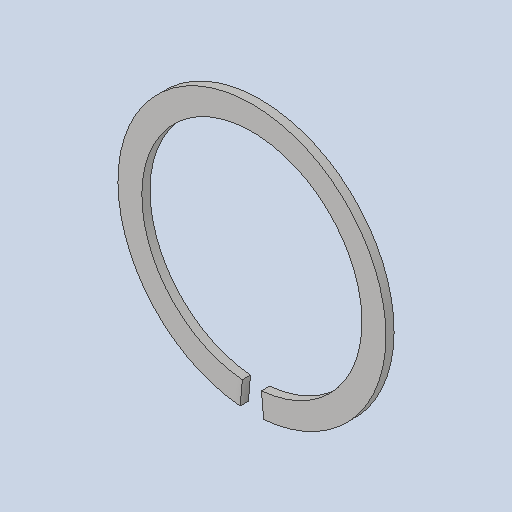
# Autodesk Inventor part: RING-6201ZZ
Saved by Autodesk Inventor 2025.1 (Build 291241000, 241)
## iProperties
Created: 2023-12-27
Part Number: RING-6201ZZ
Material: Generic
Catalog Web Link: www.cadenas.de
Description: RING-External Retaining Ring
Vendor: MISUMI
Document SubType Name: Modeling
Designer: psAdmin
Manufacturer: MISUMI
Mass: 0.374469 g
Surface Area: 9.04715 cm^2
Volume: 0.374469 cm^3
Density: 1 g/cm^3
Appearance: PSOLRGB-175-175-175
Category: PARTsolutions
Company: MISUMI
PSOL_IDENT_0: {$CADENAS_DATA/23d-libs/misumi/metric/12_bearing_holders/sb6905zznr_ring.prj},160 {VTYP=3D},{NB=RING
PSOL_IDENT_1: -6201ZZ},{LINA=RING-6201ZZ},{NN=RING},{DATE=25.04.2017 02:57:49},{GEOMDATE=03.07.2009 00:00:00},{VER
PSOL_IDENT_2: SION=},{LINEID=90},{WBVAR=},{WBNUMERIC=}  {NB=RING-6201ZZ},{LINA=RING-6201ZZ},{KT=DUMMY},{PN=RING-62
PSOL_IDENT_3: 01ZZ},{BN=6201ZZ},{D1=36.7},{FF=1.120},{D=30.150}
NB: RING-6201ZZ
NN: RING
NT: External Retaining Ring
NBSYN: $PN.
LINA: RING-6201ZZ
CATALOG: Misumi
PN: RING-6201ZZ
BN: 6201ZZ
D1: 36.7
FF: 1.12
D: 30.15
SUPPLIER: MISUMI
ARTICLENO: RING-6201ZZ
BOMINFO: RING-6201ZZ
CREATOR: CADENAS GmbH
d2: 0.000 mm
Title: RING-6201ZZ
Author: Cadenas PARTsolutions
Comments: External Retaining Ring
Autodesk Inventor part; units mm, degrees
sketch "Sketch_1" plane through (0, 0, 0) normal (0, 0, 1) x (1, 0, 0)
  arc A0 (1.5993, -18.2802) -> (-1.5993, -18.2802) centre (0, 0) ccw
  line L0 (-1.5993, -18.2802) -> (-1.3139, -15.0176)
  arc A1 (1.3139, -15.0176) -> (-1.3139, -15.0176) centre (0, 0) ccw
  line L1 (1.3139, -15.0176) -> (1.5993, -18.2802)
  constraints: 4 end point, 4 point on circle, 2 centre point
extrude "Extrusion1" add sketch "Sketch_1" along normal blind 1.12
ref_plane "ring_to_bearing_XY" through (0, 0, 0) normal (0, 0, 1) x (1, 0, 0)
ref_plane "ring_to_bearing_YZ" through (0, 0, 0) normal (1, 0, 0) x (0, 1, 0)
ref_plane "ring_to_bearing_ZX" through (0, 0, 0) normal (0, 1, 0) x (0, 0, 1)
body "Solid1"
